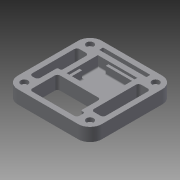
# Autodesk Inventor part: 8 pinshort
Saved by Autodesk Inventor 2015 (Build 190159000, 159)
## iProperties
Created: 2014-12-11
Part Number: 8 pinshort
Material: Generic
Document SubType Name: Modeling
Designer: Purple
Density: 1 g/cm^3
Appearance: Default
Author: Purple
Autodesk Inventor part; units mm, degrees
ref_plane "YZ Plane" through (0, 0, 0) normal (1, 0, 0) x (0, 1, 0)
ref_plane "XZ Plane" through (0, 0, 0) normal (0, 1, 0) x (-1, 0, 0)
sketch "Sketch1" plane through (0, 0, 0) normal (0, 1, 0) x (-1, 0, 0)
  line L0 (30, 30) -> (-30, 30)
  line L1 (-30, 30) -> (-30, -30)
  line L2 (-30, -30) -> (30, -30)
  line L3 (30, -30) -> (30, 30)
  line L4 (30, 30) -> (-30, -30) construction
  line L5 (-30, 30) -> (30, -30) construction
  point P0 (0, 0)
  dimension "d0" = 60
  dimension "d1" = 60
  constraints: 12 end point, 2 midpoint, 2 parallel, 1 horizontal, 1 perpendicular
  measures "d0" distance of L2.end L1.end
  measures "d1" distance of L0.end L1.end
extrude "Extrusion1" add sketch "Sketch1" along normal blind 10
fillet "Fillet1" radius 7 4 edges at (30, 5, 30) (30, 5, -30) (-30, 5, 30) (-30, 5, -30)
sketch "Sketch2" plane through (0, 10, 0) normal (0, 1, 0) x (1, 0, 0)
  line L0 (-30, 30) -> (30, 30)
  line L1 (30, 30) -> (30, -30)
  line L2 (30, -30) -> (-30, -30)
  line L3 (-30, -30) -> (-30, 30)
  line L4 (-30, 30) -> (30, -30) construction
  line L5 (30, 30) -> (-30, -30) construction
  line L6 (25, -25) -> (25, 25)
  line L7 (25, 25) -> (-25, 25)
  line L8 (-25, 25) -> (-25, -25)
  line L9 (-25, -25) -> (25, -25)
  circle A0 centre (25, -25) radius 2.75
  circle A1 centre (-25, -25) radius 2.75
  circle A2 centre (25, 25) radius 2.75
  circle A3 centre (-25, 25) radius 2.75
  point P0 (0, 0)
  dimension "d5" = 5
  dimension "d6" = 5.5
  dimension "d7" = 5.5
  dimension "d8" = 5.5
  dimension "d9" = 5.5
  constraints: 20 end point, 4 centre point, 4 coincident, 4 parallel, 2 midpoint, 2 perpendicular, 1 horizontal, 3 other
  measures "d5" distance between parallel lines of L1 L6
  measures "d6" diameter of A0
  measures "d7" diameter of A1
  measures "d8" diameter of A2
  measures "d9" diameter of A3
extrude "Extrusion2" cut sketch "Sketch2" against normal blind 3 contours L9 A0 L6 | L6 A0 L9 | A2 L7 L6 | L6 L7 A2 | A1 L8 L9 | L9 L8 A1 | A3 L8 L7 | L7 L8 A3
sketch "Sketch7" plane through (0, 10, 0) normal (0, 1, 0) x (1, 0, 0)
  line L0 (-23, 30) -> (23, 30)
  line L1 (30, 23) -> (30, -23)
  line L2 (23, -30) -> (-23, -30)
  line L3 (-30, -23) -> (-30, 23)
  line L4 (-30, 30) -> (30, -30) construction
  line L5 (30, 30) -> (-30, -30) construction
  arc A0 (-23, 30) -> (-30, 23) centre (-23, 23) ccw
  arc A1 (-30, -23) -> (-23, -30) centre (-23, -23) ccw
  arc A2 (23, -30) -> (30, -23) centre (23, -23) ccw
  arc A3 (30, 23) -> (23, 30) centre (23, 23) ccw
  line L6 (23, 32) -> (-23, 32)
  arc A4 (-23, 32) -> (-32, 23) centre (-23, 23) ccw
  line L7 (-32, 23) -> (-32, -23)
  arc A5 (-32, -23) -> (-23, -32) centre (-23, -23) ccw
  line L8 (-23, -32) -> (23, -32)
  arc A6 (23, -32) -> (32, -23) centre (23, -23) ccw
  line L9 (32, -23) -> (32, 23)
  arc A7 (32, 23) -> (23, 32) centre (23, 23) ccw
  point P0 (0, 0)
  dimension "d47" = 7
  dimension "d48" = 2
  constraints: 20 end point, 16 point on circle, 8 centre point, 8 point on line, 8 tangent, 4 parallel, 3 equal radius, 2 midpoint, 2 perpendicular, 1 horizontal, 7 other
  measures "d47" radius of A0
  measures "d48" distance between parallel lines of L0 L6
extrude "Extrusion6" add sketch "Sketch7" against normal blind 10
sketch "Sketch33" plane through (0, 10, 0) normal (0, 1, 0) x (1, 0, 0)
  line L0 (-25, 25) -> (25, 25)
  line L1 (25, 25) -> (25, -25)
  line L2 (25, -25) -> (-25, -25)
  line L3 (-25, -25) -> (-25, 25)
  line L4 (-25, 25) -> (25, -25) construction
  line L5 (25, 25) -> (-25, -25) construction
  line L6 (21, 21) -> (-21, 21)
  line L7 (-21, 21) -> (-21, -21)
  line L8 (-21, -21) -> (21, -21)
  line L9 (21, -21) -> (21, 21)
  line L10 (-15, 21) -> (-15, -2.8)
  line L11 (-15, -2.8) -> (15, -2.8)
  line L12 (15, -2.8) -> (15, 21)
  line L13 (-13, 7) -> (-13, -0.8)
  line L14 (-13, -0.8) -> (6, -0.8)
  line L15 (13, -0.8) -> (13, 19)
  line L16 (-7, 21) -> (-7, 19)
  line L17 (-7, 19) -> (13, 19)
  line L18 (13, -0.8) -> (13, -2.8)
  line L19 (6, -2.8) -> (6, -0.8)
  line L20 (-15, 7) -> (-13, 7)
  point P0 (0, 0)
  point P1 (-21, 15)
  dimension "d349" = 50
  dimension "d350" = 50
  dimension "d351" = 4
  dimension "d352" = 6
  dimension "d353" = 30
  dimension "d354" = 6
  dimension "d355" = 23.8
  dimension "d356" = 8
  dimension "d357" = 2
  dimension "d358" = 7
  dimension "d359" = 2
  dimension "d360" = 2
  dimension "d361" = 14
  constraints: 42 end point, 9 perpendicular, 7 point on line, 4 parallel, 2 midpoint, 2 vertical, 1 horizontal, 3 other
  measures "d349" distance of L1.end L2.end
  measures "d350" distance of L0.end L1.end
  measures "d351" distance between parallel lines of L0 L6
  measures "d352" distance of L10.start L6.end
  measures "d353" distance of L10.start L12.end
  measures "d354" horizontal distance of point (-21, 15) L10.start
  measures "d355" distance of L10.start L10.end
  measures "d356" distance of L16.start L10.start
  measures "d357" distance of L11.end L18.end
  measures "d358" distance of L18.end L19.start
  measures "d359" distance between parallel lines of L10 L13
  measures "d360" distance of L16.end L16.start
  measures "d361" distance of L20.start L10.start
extrude "Extrusion31" cut sketch "Sketch33" against normal blind 2 contours L12 L11 L18 L15 L17 L16 L6 | L20 L13 L14 L19 L11 L10
sketch "Sketch34" plane through (0, 10, 0) normal (0, 1, 0) x (1, 0, 0)
  line L0 (13, -2.8) -> (6, -2.8)
  line L1 (6, -2.8) -> (6, -0.8)
  line L2 (6, -0.8) -> (-13, -0.8)
  line L3 (-13, -0.8) -> (-13, 7)
  line L4 (-13, 7) -> (-15, 7)
  line L5 (-15, 7) -> (-15, 21)
  line L6 (-15, 21) -> (-7, 21)
  line L7 (-7, 21) -> (-7, 19)
  line L8 (-7, 19) -> (13, 19)
  line L9 (13, 19) -> (13, -2.8)
  line L10 (13, -2.8) -> (13, 19) projected
  point P0 (0, 0)
  constraints: 20 end point, 8 perpendicular, 1 collinear, 1 horizontal
extrude "Extrusion32" cut sketch "Sketch34" against normal blind 8
sketch "Sketch35" plane through (0, 10, 0) normal (0, 1, 0) x (1, 0, 0)
  line L0 (23, 32) -> (-23, 32) projected
  line L1 (-32, 23) -> (-32, -23) projected
  line L2 (32, -23) -> (32, 23) projected
  line L3 (-15, 21) -> (15, 21) projected
  line L4 (18, 28) -> (-18, 28)
  line L5 (-18, 28) -> (-18, 25)
  line L6 (-18, 25) -> (18, 25)
  line L7 (18, 25) -> (18, 28)
  line L8 (-23, -32) -> (23, -32) projected
  line L9 (15, 21) -> (15, -2.8) projected
  line L10 (28, -18) -> (28, 18)
  line L11 (28, 18) -> (19, 18)
  line L12 (19, 18) -> (19, -18)
  line L13 (19, -18) -> (28, -18)
  line L14 (15, -2.8) -> (-15, -2.8) projected
  line L15 (-18, -28) -> (18, -28)
  line L16 (18, -28) -> (18, -22)
  line L17 (18, -22) -> (15, -22)
  line L18 (15, -22) -> (15, -6.8)
  line L19 (15, -6.8) -> (-18, -6.8)
  line L20 (-18, -6.8) -> (-18, -28)
  line L21 (-15, -2.8) -> (-15, 21) projected
  line L22 (-22, -18) -> (-28, -18)
  line L23 (-28, -18) -> (-28, 18)
  line L24 (-28, 18) -> (-19, 18)
  line L25 (-19, 18) -> (-19, -2.8)
  line L26 (-19, -2.8) -> (-22, -2.8)
  line L27 (-22, -2.8) -> (-22, -18)
  point P0 (0, 0)
  dimension "d366" = 4
  dimension "d367" = 4
  dimension "d368" = 14
  dimension "d369" = 14
  dimension "d370" = 4
  dimension "d371" = 4
  dimension "d372" = 14
  dimension "d373" = 4
  dimension "d374" = 14
  dimension "d375" = 4
  dimension "d376" = 4
  dimension "d377" = 14
  dimension "d378" = 4
  dimension "d379" = 4
  dimension "d380" = 4
  dimension "d381" = 14
  dimension "d382" = 4
  dimension "d383" = 14
  dimension "d384" = 14
  dimension "d385" = 4
  dimension "d386" = 4
  dimension "d387" = 4
  constraints: 40 end point, 14 perpendicular, 1 horizontal, 1 parallel
  measures "d366" distance from line of L4.end L0
  measures "d367" distance from line of L0 L4.start
  measures "d368" distance from line of L1 L4.end
  measures "d369" distance from line of L2 L4.start
  measures "d370" distance from line of L5.end L3
  measures "d371" distance from line of L10.end L2
  measures "d372" distance from line of L0 L10.end
  measures "d373" distance from line of L2 L10.start
  measures "d374" distance from line of L10.start L8
  measures "d375" distance from line of L11.end L9
  measures "d376" distance from line of L8 L15.end
  measures "d377" distance from line of L2 L15.end
  measures "d378" distance from line of L16.end L13
  measures "d379" distance from line of L18.end L14
  measures "d380" distance from line of L8 L15.start
  measures "d381" distance from line of L1 L15.start
  measures "d382" distance from line of L1 L23.end
  measures "d383" distance from line of L0 L23.end
  measures "d384" distance from line of L8 L22.end
  measures "d385" distance from line of L1 L22.end
  measures "d386" distance from line of L21 L24.end
  measures "d387" distance from line of L22.start L20
extrude "Extrusion33" cut sketch "Sketch35" against normal through all contours L7 L6 L5 L4 | L13 L12 L11 L10 | L20 L19 L18 L17 L16 L15 | L22 L23 L24 L25 L26 L27
fillet "Fillet10" radius 2 12 edges at (19, 5, 18) (-28, 5, 18) (-18, 5, 28) (15, 5, 6.8) (28, 5, -18) (28, 5, 18) (18, 5, 28) (-18, 5, 6.8) (19, 5, -18) (-28, 5, -18) (-19, 5, -18) (-22, 5, 18)
fillet "Fillet10" radius 1 14 edges at (15, 5, 22) (9.5, 2, 2.8) (13, 2, -8.1) (-3.5, 2, 0.8) (-13, 2, -3.1) (-15, 2, -14) (-22, 5, 2.8) (-19, 5, 2.8) (18, 5, 22) (3, 2, -19) (-11, 2, -21) (-14, 2, -7) (6, 2, 1.8) (-7, 2, -20)
fillet "Fillet10" radius 0.5 4 edges at (-18, 5, -25) (-18, 5, -28) (18, 5, -25) (18, 5, -28)
ref_plane "Work Plane9" through (0, 5, 0) normal (0, 1, 0) x (1, 0, 0)
mirror "Mirror9" about plane through (0, 5, 0) normal (0, 1, 0) of "Extrusion2"
body "Solid1"
